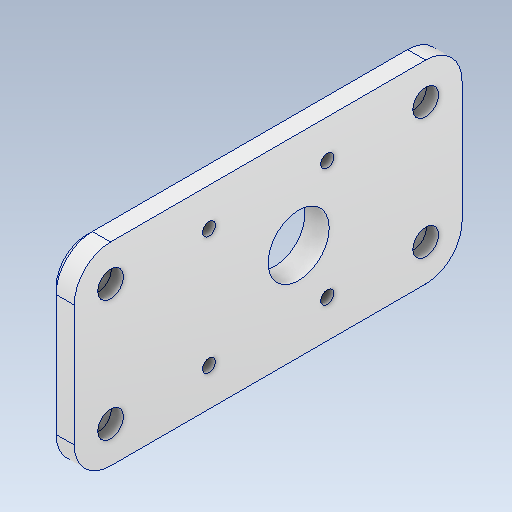
# Autodesk Inventor part: NASA-20-MM-MP-01
Saved by Autodesk Inventor 2020 (Build 240168000, 168)
## iProperties
Created: 2019-09-22
Part Number: NASA-20-MM-MP-01
Material: Aluminum 6061
Document SubType Name: Modeling
Designer: Rick Szalay
Density: 2.7 g/cm^3
Appearance: Aluminum - Flat
Description: MOUNTING PLATE, MOTOR
Author: Rick Szalay
Autodesk Inventor part; units mm, degrees
ref_plane "YZ Plane" through (0, 0, 0) normal (1, 0, 0) x (0, 1, 0)
ref_plane "XZ Plane" through (0, 0, 0) normal (0, 1, 0) x (-1, 0, 0)
ref_plane "XY Plane" through (0, 0, 0) normal (0, 0, 1) x (1, 0, 0)
sketch "Sketch1" plane through (0, 0, 0) normal (1, 0, 0) x (0, 1, 0)
  line L0 (-25.4, 50.8) -> (25.4, 50.8)
  line L1 (25.4, 50.8) -> (25.4, -50.8)
  line L2 (25.4, -50.8) -> (-25.4, -50.8)
  line L3 (-25.4, -50.8) -> (-25.4, 50.8)
  line L4 (-25.4, 50.8) -> (25.4, -50.8) construction
  line L5 (25.4, 50.8) -> (-25.4, -50.8) construction
  point P0 (0, 0)
  dimension "d0" = 50.8
  dimension "d1" = 101.6
  constraints: 12 end point, 2 midpoint, 2 parallel, 1 horizontal, 1 perpendicular
  measures "d0" distance of L1.end L2.end
  measures "d1" distance of L0.end L1.end
extrude "Extrusion1" add sketch "Sketch1" along normal blind 6.35
fillet "Fillet1" radius 9.525 4 edges at (3.175, 25.4, 50.8) (3.175, -25.4, 50.8) (3.175, -25.4, -50.8) (3.175, 25.4, -50.8)
sketch "Sketch2" plane through (0, 0, 0) normal (-1, 0, 0) x (0, 0, 1)
  circle A0 centre (-8, 0) radius 8 projected
  point P0 (0, 0)
  dimension "d5" = 16
  constraints: 1 horizontal alignment
extrude "Extrusion2" cut sketch "Sketch2" against normal through all
sketch "Sketch3" plane through (0, 0, 0) normal (-1, 0, 0) x (0, 0, 1)
  circle A0 centre (-8, 0) radius 8 projected
  arc A1 (-41.275, 25.4) -> (-50.8, 15.875) centre (-41.275, 15.875) ccw projected
  line L0 (-50.8, -15.875) -> (-50.8, 15.875) projected
  arc A2 (-50.8, -15.875) -> (-41.275, -25.4) centre (-41.275, -15.875) ccw projected
  line L1 (41.275, -25.4) -> (-41.275, -25.4) projected
  arc A3 (41.275, -25.4) -> (50.8, -15.875) centre (41.275, -15.875) ccw projected
  line L2 (50.8, 15.875) -> (50.8, -15.875) projected
  arc A4 (50.8, 15.875) -> (41.275, 25.4) centre (41.275, 15.875) ccw projected
  line L3 (-41.275, 25.4) -> (41.275, 25.4) projected
  point P0 (0, 0)
hole "Hole1" at (0, 15.875, -41.275) at (0, -15.875, -41.275) at (0, -15.875, 41.275) at (0, 15.875, 41.275) direction (1, 0, 0) diameter 6.7564 end through all counterbore diameter 11.1252 counterbore depth 3.175 clearance for "Socket Head Cap Screw" size "1/4" standard "Ansi Unified Screw Threads"
chamfer "Chamfer1" distance 1.5875 angle 45 8 edges at (0, 0, -50.8) (0, 22.6102, -48.0102) (0, 25.4, 0) (0, 22.6102, 48.0102) (0, 0, 50.8) (0, -22.6102, 48.0102) (0, -25.4, 0) (0, -22.6102, -48.0102)
sketch "Sketch4" plane through (0, 0, 0) normal (-1, 0, 0) x (0, 0, 1)
  circle A0 centre (15.4856, 15.4856) radius 1.621 projected
  circle A1 centre (-15.4856, 15.4856) radius 1.621 projected
  circle A2 centre (-15.4856, -15.4856) radius 1.621 projected
  circle A3 centre (15.4856, -15.4856) radius 1.621 projected
  point P0 (0, 0)
hole "Hole2" at (0, 15.4856, -15.4856) at (0, 15.4856, 15.4856) at (0, -15.4856, 15.4856) at (0, -15.4856, -15.4856) direction (1, 0, 0) diameter 3.4036 end through all counterbore diameter 6.5024 counterbore depth 3.4036 clearance for "Socket Head Cap Screw DIN EN ISO 4762" size "M3" standard "DIN"
body "Solid1"
